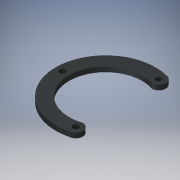
# Autodesk Inventor part: Revers Lever Ring
Saved by Autodesk Inventor 2017 (Build 210142000, 142)
## iProperties
Created: 2018-11-02
Part Number: Revers Lever Ring
Material: Iron, Gray
Document SubType Name: Modeling
Designer: 623516
Density: 7.15 g/cm^3
Appearance: Iron Gray
Author: 623516
Autodesk Inventor part; units mm, degrees
ref_plane "YZ Plane" through (0, 0, 0) normal (1, 0, 0) x (0, 1, 0)
ref_plane "XZ Plane" through (0, 0, 0) normal (0, 1, 0) x (-1, 0, 0)
ref_plane "XY Plane" through (0, 0, 0) normal (0, 0, 1) x (1, 0, 0)
sketch "Sketch1" plane through (0, 0, 0) normal (0, 1, 0) x (-1, 0, 0)
  circle A0 centre (0, 0) radius 30 construction
  circle A1 centre (0, 0) radius 22 construction
  line L0 (0, 0) -> (-7, 0) construction
  line L1 (-7, 0) -> (-7, 79.693) construction
  line L2 (-7, 0) -> (-7, -62.3337) construction
  arc A2 (-7, -20.8567) -> (-7, 20.8567) centre (0, 0) ccw
  arc A3 (-7, -29.1719) -> (-7, 29.1719) centre (0, 0) ccw
  line L3 (-7, -20.8567) -> (-7, -29.1719) construction
  circle A4 centre (-7, -25.0143) radius 1.75 construction
  line L4 (-7, 29.1719) -> (-7, 20.8567) construction
  circle A5 centre (-7, 25.0143) radius 1.75 construction
  circle A6 centre (-7, 25.0143) radius 4.1576 construction
  arc A7 (-7, 29.1719) -> (-7, 20.8567) centre (-7, 25.0143) ccw construction
  circle A8 centre (-7, 25.0143) radius 1.75
  arc A9 (-7, 29.1719) -> (-7, 20.8567) centre (-7, 25.0143) ccw
  circle A10 centre (-7, -25.0143) radius 1.75
  circle A11 centre (-7, -25.0143) radius 4.1576 construction
  arc A12 (-7, -20.8567) -> (-7, -29.1719) centre (-7, -25.0143) ccw
  line L5 (22, 0) -> (30, 0) construction
  circle A13 centre (26, 0) radius 1.75
  dimension "d0" = 60
  dimension "d1" = 8
  dimension "d3" = 7
  dimension "d4" = 3.5
  dimension "d5" = 3.5
  dimension "d8" = 3.5
  constraints: 16 point on circle, 12 centre point, 12 end point, 10 coincident, 6 concentric, 4 point on line, 3 midpoint, 2 collinear, 2 vertical alignment, 1 horizontal, 1 perpendicular, 1 vertical, 10 other
  measures "d0" diameter of A0
  measures "d1" radial gap between concentric circles of A0 A1
  measures "d3" distance of L0.start L0.end
  measures "d4" diameter of A4
  measures "d5" diameter of A5
  measures "d8" diameter of A13
extrude "Extrusion2" add sketch "Sketch1" along normal blind 3
body "Solid2"
